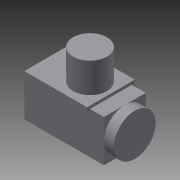
# Autodesk Inventor part: Wrist_Yaw
Saved by Autodesk Inventor 2013 (Build 170138000, 138)
## iProperties
Created: 2012-12-04
Part Number: Wrist_Yaw
Material: Generic
Document SubType Name: Modeling
Designer: Joe
Density: 1 g/cm^3
Author: Joe
Autodesk Inventor part; units mm, degrees
ref_plane "YZ Plane" through (0, 0, 0) normal (1, 0, 0) x (0, 1, 0)
ref_plane "XZ Plane" through (0, 0, 0) normal (0, 1, 0) x (-1, 0, 0)
ref_plane "XY Plane" through (0, 0, 0) normal (0, 0, 1) x (1, 0, 0)
sketch "Sketch1" plane through (0, 0, 0) normal (0, 1, 0) x (-1, 0, 0)
  circle A0 centre (0, 0) radius 17
  dimension "d0" = 34
  constraints: 1 centre point, 1 coincident
  measures "d0" diameter of A0
extrude "Extrusion1" add sketch "Sketch1" against normal blind 30
sketch "Sketch2" plane through (0, -30, 0) normal (0, -1, 0) x (1, 0, 0)
  circle A0 centre (0, 0) radius 17 projected
  line L0 (0, 0) -> (0, -21) construction
  line L1 (0, 0) -> (-24, 0) construction
  line L2 (0, -21) -> (-24, -21)
  line L3 (-24, 0) -> (-24, -21)
  line L4 (0, -21) -> (24, -21)
  line L5 (24, 0) -> (24, -21)
  line L6 (0, 21) -> (-24, 21)
  line L7 (-24, 0) -> (-24, 21)
  line L8 (0, 21) -> (24, 21)
  line L9 (24, 0) -> (24, 21)
  dimension "d5" = 21
  dimension "d6" = 24
  constraints: 20 end point, 5 symmetric about line, 2 perpendicular, 1 parallel, 1 vertical
  measures "d5" distance of L0.start L0.end
  measures "d6" distance of L0.start L1.end
extrude "Extrusion2" add sketch "Sketch2" along normal blind 6 contours A0 | L2 L3 L7 L6 L8 L9 L5 L4
sketch "Sketch3" plane through (-24, -30, 21) normal (0, 0, 1) x (1, 0, 0)
  line L0 (0, 0) -> (48, 0) projected
  line L1 (48, -6) -> (0, -6) projected
  line L2 (3, -6) -> (45, -6)
  line L3 (45, -6) -> (45, -3)
  line L4 (45, -3) -> (3, -3)
  line L5 (3, -3) -> (3, -6)
  line L6 (24, 0) -> (24, -6) construction
  line L7 (24, -3) -> (24, -6) construction
  point P0 (24, 30)
  dimension "d9" = 3
  dimension "d11" = 42
  constraints: 12 end point, 4 midpoint, 2 parallel, 2 perpendicular, 1 collinear, 1 horizontal, 1 point on line
  measures "d9" distance of L4.end L2.start
  measures "d11" distance of L3.end L4.end
extrude "Extrusion3" cut sketch "Sketch3" against normal through all
sketch "Sketch4" plane through (0, 0, 0) normal (0, 0, 1) x (1, 0, 0)
  line L0 (-21, -33) -> (21, -33)
  line L1 (21, -33) -> (21, -75)
  line L2 (21, -75) -> (-21, -75)
  line L3 (-21, -75) -> (-21, -33)
  line L4 (-21, -36) -> (-21, -33) projected
  line L5 (-21, -33) -> (21, -33) projected
  line L6 (21, -33) -> (21, -36) projected
  point P0 (0, 0)
  constraints: 8 end point, 3 collinear, 2 parallel, 2 perpendicular, 1 horizontal
extrude "Extrusion4" add sketch "Sketch4" along normal mid plane 90
sketch "Sketch5" plane through (0, 0, 45) normal (0, 0, 1) x (1, 0, 0)
  line L0 (21, -33) -> (-21, -33) projected
  line L1 (-21, -33) -> (-21, -75) projected
  line L2 (-21, -75) -> (21, -75) projected
  line L3 (21, -75) -> (21, -33) projected
  line L4 (-21, -33) -> (21, -75) construction
  circle A0 centre (0, -54) radius 21
  point P0 (0, 0)
  constraints: 2 end point, 1 centre point, 1 midpoint
extrude "Extrusion5" cut sketch "Sketch5" against normal blind 10 contours L3 A0 L0 | A0 L1 L0 | L3 L2 A0 | A0 L2 L1
move or copy body "Move Body1" bodies to move or copy 1 copy no rotation origin (0, 0, 0) rotation axis (1, 0, 0) rotation angle 90
move or copy body "Move Body2" bodies to move or copy 1 copy no rotation origin (0, 0, 0) rotation axis (0, 0, 1) rotation angle 90
move or copy body "Move Body3" bodies to move or copy 1 copy no translate (0, 0, 54)
body "Solid1"
